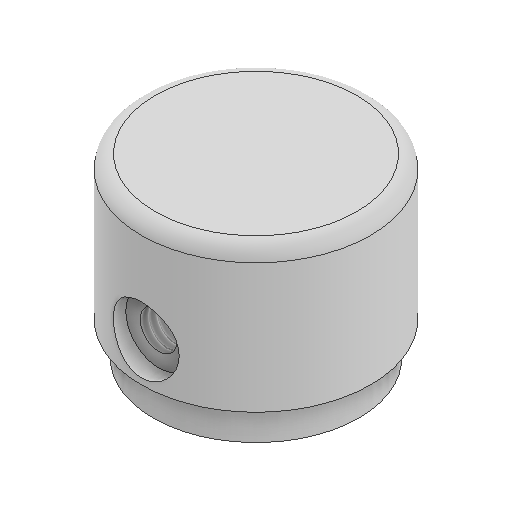
# Autodesk Inventor part: encoder_cap
Saved by Autodesk Inventor 2025 (Build 290162000, 162)
## iProperties
Created: 2025-01-07
Part Number: encoder_cap
Material: Generic
Document SubType Name: Modeling
Designer: Jan Mareš
Density: 1 g/cm^3
Appearance: Default
Author: Jan Mareš
Autodesk Inventor part; units mm, degrees
note: some values were not read from the file. Chosen so that the rebuilt part matches the saved one: direction of "Hole1".
ref_plane "YZ Plane" through (0, 0, 0) normal (1, 0, 0) x (0, 1, 0)
ref_plane "XZ Plane" through (0, 0, 0) normal (0, 1, 0) x (-1, 0, 0)
sketch "Sketch1" plane through (0, 0, 0) normal (0, 0, 1) x (1, 0, 0)
  line L0 (0, -3.1) -> (0, 18.6) construction
  line L1 (-2, 0) -> (12, 0) construction
  line L2 (9, 0) -> (9, 3)
  line L3 (9, 3) -> (10, 3)
  line L4 (10, 3) -> (10, 15.5)
  line L5 (10, 15.5) -> (0, 15.5)
  line L6 (0, 15.5) -> (0, 12)
  line L7 (0, 12) -> (3, 12)
  line L8 (3, 12) -> (3, 3)
  line L9 (3, 3) -> (7.5, 3)
  line L10 (7.5, 3) -> (7.5, 0)
  line L11 (7.5, 0) -> (9, 0)
  point P0 (0, 0)
  point P1 (3, 7.5)
  dimension "d0" = 15.5
  dimension "d1" = 12
  dimension "d2" = 3
  dimension "d4" = 6
  dimension "d5" = 15
  dimension "d6" = 18
  dimension "d7" = 20
  constraints: 20 end point, 6 point on line, 5 perpendicular, 1 collinear, 1 horizontal, 1 midpoint, 1 vertical
  measures "d0" distance between parallel lines of L1 L5
  measures "d1" distance between parallel lines of L1 L7
  measures "d2" distance between parallel lines of L1 L3
  measures "d4" diameter of L8 L0
  measures "d5" diameter of L10 L0
  measures "d6" diameter of L2 L0
  measures "d7" diameter of L4 L0
revolve "Revolution1" add sketch "Sketch1" angle 360 about axis through (0, -10, 0) along (0, 1, 0)
fillet "Fillet1" radius 1.2 1 edges at (-10, 15.5, 0)
ref_plane "Work Plane1" through (0, 9.25, 10) normal (0, 0, 1) x (1, 0, 0)
sketch "Sketch3" plane through (0, 9.25, 10) normal (0, 0, 1) x (1, 0, 0)
  line L0 (9, -9.25) -> (-9, -9.25) construction
  line L1 (0, -12.35) -> (0, 9.35) construction
  point P0 (0, -9.25)
  point P1 (0, -2.85)
  dimension "d11" = 6.4
  constraints: 1 point on line
  measures "d11" distance from line of L0 point (0, -2.85)
hole "Hole1" at (0, 6.4, 10) direction (0, 0, -1) diameter 3.242 end up to surface counterbore diameter 5.75 counterbore depth 1.5 thread size "M4x0.7" class "6H" standard "ISO Metric profile"
body "Solid1"
